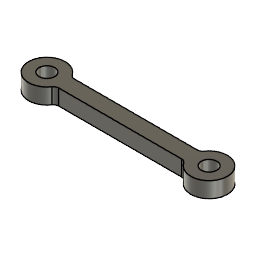
GripperP2 (Autodesk Fusion 360 design; units mm, degrees)
part number: 2026-06-13-13-05-51-409
Autodesk Fusion 360 part; units mm, degrees
note: some values were not read from the file. Set by a fixed rule: which sketch regions a step uses.
sketch "Sketch1" plane through (0, 0, 0) normal (0, 0, 1) x (1, 0, 0)
  circle A0 centre (30.6182, 28.8633) radius 1.5
  circle A1 centre (30.6182, 28.8633) radius 3.5
  circle A2 centre (61.6182, 28.8633) radius 1.5
  circle A3 centre (61.6182, 28.8633) radius 3.5
  line L0 (30.6182, 28.8633) -> (61.6182, 28.8633)
  line L1 (33.7805, 30.3633) -> (59, 30.3633)
  line L2 (33.7805, 27.3633) -> (59, 27.3633)
  dimension "d1" = 3
  dimension "d2" = 7
  dimension "d3" = 3
  dimension "d4" = 7
  dimension "d5" = 31
  dimension "d6" = 1.5
  constraint concentric A0 A1
  constraint concentric A2 A3
  constraint coincident A0.centre A1.centre
  constraint coincident A2.centre A3.centre
  constraint horizontal L0
  constraint coincident A1 L1.start
  constraint horizontal L1
  constraint symmetric L0 L1.start L2.start
  constraint symmetric L0 L1.end L2.end
  measures "d1" diameter of A0
  measures "d2" diameter of A1
  measures "d3" diameter of A2
  measures "d4" diameter of A3
  measures "d5" distance of A0.centre A2.centre
  measures "d6" distance of L0 L1
extrude "Extrude1" add sketch "Sketch1" along normal blind 3
fillet "Fillet1" radius 1 4 edges at (33.7805, 30.3633, 1.5) (58.456, 30.3633, 1.5) (33.7805, 27.3633, 1.5) (58.456, 27.3633, 1.5)
